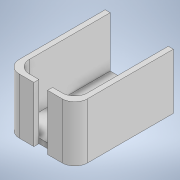
# Autodesk Inventor part: Hộp đựng động cơ
Saved by Autodesk Inventor 2020 (Build 240168000, 168)
## iProperties
Created: 2022-04-01
Part Number: Hộp đựng động cơ
Material: Generic
Document SubType Name: Modeling
Designer: PC
Density: 1 g/cm^3
Appearance: Default
Author: PC
Autodesk Inventor part; units mm, degrees
ref_plane "YZ Plane" through (0, 0, 0) normal (1, 0, 0) x (0, 1, 0)
ref_plane "XZ Plane" through (0, 0, 0) normal (0, 1, 0) x (-1, 0, 0)
ref_plane "XY Plane" through (0, 0, 0) normal (0, 0, 1) x (1, 0, 0)
sketch "Sketch1" plane through (0, 0, 0) normal (0, 1, 0) x (-1, 0, 0)
  line L0 (0, 0) -> (-27, 0)
  line L1 (-27, 0) -> (-27, -39)
  line L2 (-27, -39) -> (0, -39)
  line L3 (0, -39) -> (0, 0)
  dimension "d0" = 27
  dimension "d1" = 39
  constraints: 8 end point, 2 parallel, 1 horizontal, 1 perpendicular
  measures "d0" distance of L2.end L1.end
  measures "d1" distance of L0.end L1.end
extrude "Extrusion1" add sketch "Sketch1" along normal blind 22
sketch "Sketch2" plane through (0, 22, 0) normal (0, 1, 0) x (1, 0, 0)
  line L0 (27, 39) -> (0, 39) projected
  line L1 (2, 39) -> (2, 2)
  line L2 (2, 2) -> (25, 2)
  line L3 (25, 2) -> (25, 39)
  line L4 (27, 0) -> (27, 39) projected
  line L5 (0, 39) -> (0, 0) projected
  line L6 (0, 0) -> (27, 0) projected
  dimension "d4" = 2
  dimension "d5" = 2
  dimension "d6" = 2
  constraints: 6 end point, 2 perpendicular, 2 point on line, 1 vertical
  measures "d4" distance between parallel lines of L4 L3
  measures "d5" distance between parallel lines of L1 L5
  measures "d6" distance between parallel lines of L6 L2
extrude "Extrusion2" cut sketch "Sketch2" against normal blind 20 contours L3 L2 L1 L0
fillet "Fillet1" radius 5 4 edges at (27, 11, 0) (0, 11, 0) (2, 12, -2) (25, 12, -2)
sketch "Sketch3" plane through (0, 2, 0) normal (0, 1, 0) x (1, 0, 0)
  circle A0 centre (13.5, 13.2) radius 2.75
  line L0 (20, 2) -> (7, 2) projected
  point P0 (0, 0)
  dimension "d10" = 5.5
  dimension "d11" = 11.2
  constraints: 1 centre point
  measures "d10" diameter of A0
  measures "d11" distance from line of L0 A0.centre
extrude "Extrusion3" cut sketch "Sketch3" against normal through all
sketch "Sketch5" plane through (0, 22, 0) normal (0, 1, 0) x (1, 0, 0)
  line L0 (5, 0) -> (22, 0) projected
  line L1 (13.5, 0) -> (13.5, 2)
  line L2 (20, 2) -> (7, 2) projected
  line L3 (10.8, 0) -> (16.2, 0)
  line L4 (16.2, 0) -> (16.2, 2)
  line L5 (16.2, 2) -> (10.8, 2)
  line L6 (10.8, 2) -> (10.8, 0)
  line L7 (10.8, 0) -> (16.2, 2) construction
  line L8 (16.2, 0) -> (10.8, 2) construction
  point P0 (0, 0)
  point P1 (13.5, 1)
  dimension "d17" = 5.4
  constraints: 14 end point, 5 midpoint, 2 parallel, 1 horizontal, 1 perpendicular, 1 point on line
  measures "d17" distance of L5.end L4.end
extrude "Extrusion4" cut sketch "Sketch5" against normal through all
body "Solid1"
